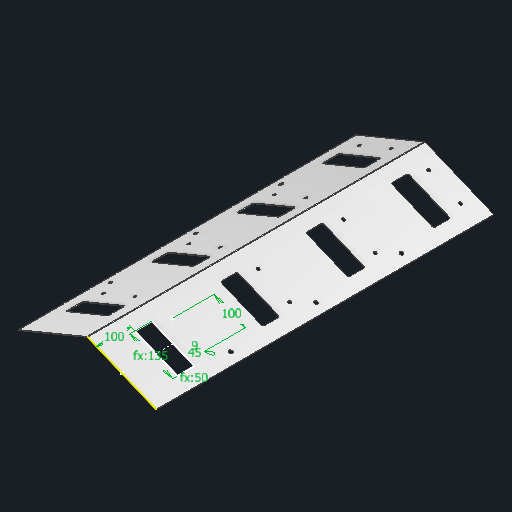
# Autodesk Inventor part: ASY DMF 010 cap №2 v2.1
Saved by Autodesk Inventor 2026.2 (Build 302298010, 298A)
## iProperties
Created: 2024-04-28
Part Number: ASY DMF 010 cap №2 v2.1
Material: Stainless Steel AISI 304
Document SubType Name: Sheet Metal
Designer: pokla
Stock Number: Барабан_Лист_Крышка
Density: 8 g/cm^3
Flat Pattern Width: 43.6215 cm
Flat Pattern Length: 98.85 cm
Flat Pattern Area: 4311.98 cm^2
Sheet Metal Rule: Default
Sheet Metal Width: 436,215 mm
Sheet Metal Length: 988,500 mm
Sheet Metal Area: 431198,146 mm^2
Appearance: Chrome - Satin
Author: pokla
Autodesk Inventor part; units mm, degrees
note: some values were not read from the file. Chosen so that the rebuilt part matches the saved one: flange form of "Plate4".
ref_plane "YZ Plane" through (0, 0, 0) normal (1, 0, 0) x (0, 1, 0)
ref_plane "XZ Plane" through (0, 0, 0) normal (0, 1, 0) x (-1, 0, 0)
ref_plane "XY Plane" through (0, 0, 0) normal (0, 0, 1) x (1, 0, 0)
sketch "Sketch1" plane through (0, 0, 0) normal (0, 0, 1) x (1, 0, 0)
  line L0 (-202.822219, 202.822219) -> (0, 286.833933) construction
  line L1 (0, 286.833933) -> (202.822219, 202.822219) construction
  line L2 (202.822219, 202.822219) -> (286.833933, 0) construction
  line L3 (286.833933, 0) -> (202.822219, -202.822219) construction
  line L4 (202.822219, -202.822219) -> (0, -286.833933) construction
  line L5 (0, -286.833933) -> (-202.822219, -202.822219) construction
  line L6 (-202.822219, -202.822219) -> (-286.833933, 0) construction
  line L7 (-286.833933, 0) -> (-202.822219, 202.822219) construction
  line L8 (1.530734, 286.199882) -> (201.990728, 203.166634)
  line L9 (-1.530734, 286.199882) -> (-201.990728, 203.166634)
  arc A0 (1.530734, 286.199882) -> (-1.530734, 286.199882) centre (0, 282.504364) ccw
  point P0 (0, 0)
  point P1 (0, 0)
  dimension "d46" = 530
  dimension "d47" = 0.9
  dimension "d48" = 4
  measures "d46" distance between parallel lines of L7 L3
  measures "d47" distance of L0.start L9.end
  measures "d48" radius of A0
contour flange "Contour Flange2" sketch "Sketch1" thickness 2 bend radius 2 width 988.5 along (0, 0, -1) mid plane no both sides no wall seen from (101.760731, 244.683258, 0) lies toward (-0.3826834, -0.9238795, 0) curves L8 A0 L9
bend "Bend4"
corner "Corner4"
sketch "Sketch14" plane through (1.530734, 286.199882, 0) normal (0.3826834, 0.9238795, 0) x (0.9238795, -0.3826834, 0)
  line L0 (175.988167, 150) -> (175.988167, 100)
  line L1 (175.988167, 100) -> (40.988167, 100)
  line L2 (40.988167, 100) -> (40.988167, 150)
  line L3 (40.988167, 150) -> (175.988167, 150)
  circle A0 centre (158.488167, 195) radius 4.5
  circle A1 centre (58.488167, 195) radius 4.5
  line L4 (108.488167, 100) -> (108.488167, 150) construction
  line L5 (216.976334, 0) -> (0, 0)
  point P0 (108.488167, 0)
  dimension "d163" = 9
  dimension "d164" = 135
  dimension "d165" = 50
  dimension "d166" = 45
  dimension "d167" = 100
  dimension "d171" = 100
  constraints: 10 end point, 3 midpoint, 2 centre point, 2 parallel, 1 perpendicular, 1 vertical alignment, 1 other
  measures "d163" diameter of A0
  measures "d164" distance of L2.end L0.start
  measures "d165" distance of L0.start L0.end
  measures "d166" distance from line of A0.centre L3
  measures "d167" distance of A1.centre A0.centre
  measures "d171" distance between parallel lines of L5 L1
extrude "Cut2" cut sketch "Sketch14" against normal through all
fillet "Fillet3" radius 5 4 edges at (39.0162, 269.5905, -150) (39.0162, 269.5905, -100) (163.7399, 217.9282, -100) (163.7399, 217.9282, -150)
pattern_linear "Rectangular Pattern7" count 4 spacing 250 along (0, 0, -1) of "Cut2", "Fillet3"
pattern_circular "Circular Pattern2" count 2 over 45 about axis through (0, 0, -10) along (0, 0, 1) of "Cut2", "Fillet3", "Rectangular Pattern7"
sketch "Sketch12" plane through (1.530734, 286.199882, 0) normal (0.3826834, 0.9238795, 0) x (0.9238795, -0.3826834, 0)
  circle A0 centre (189.129, 40.75) radius 5.5
  line L0 (0, 0) -> (0, 988.5)
  line L1 (216.976334, 0) -> (0, 0)
  line L2 (216.976334, 988.5) -> (0, 988.5)
  point P0 (108.10974, 0)
  dimension "d115" = 11
  dimension "d116" = 189.129
  dimension "d117" = 40.75
  constraints: 1 centre point
  measures "d115" diameter of A0
  measures "d116" distance from line of L0 A0.centre
  measures "d117" distance from line of L1 A0.centre
extrude "Extrusion5" [suppressed]
sketch "Sketch15" plane through (1.530734, 286.199882, 0) normal (0.3826834, 0.9238795, 0) x (0.9238795, -0.3826834, 0)
  circle A0 centre (189.129, 494.25) radius 5.5
  line L0 (0, 0) -> (0, 988.5) projected
  point P0 (108.10974, 0)
  point P1 (0, 494.25)
  dimension "d146" = 11
  dimension "d147" = 189.129
  constraints: 1 centre point, 1 horizontal alignment, 1 midpoint
  measures "d146" diameter of A0
  measures "d147" distance from line of L0 A0.centre
extrude "Extrusion8" cut sketch "Sketch15" against normal through all
pattern_linear "Rectangular Pattern6" count 3 spacing 250 along (0, 0, 1) of "Extrusion8" first direction both ways yes
mirror "Mirror5" about plane through (0, 0, 0) normal (1, 0, 0) of "Extrusion8", "Rectangular Pattern6"
equation "\"d46\" = Барабан_размер_по_плоскостям"
equation "\"d47\" = Барабан_отступ_развертки"
equation "\"d48\" = BendRadius + Thickness"
equation "\"d49\" = Thickness"
equation "\"d50\" = BendReliefWidth"
equation "\"d51\" = BendReliefDepth"
equation "\"d52\" = MinimumRemnant"
equation "\"d53\" = TransitionRadius"
equation "\"d55\" = BendRadius"
equation "\"d57\" = CornerReliefSize"
equation "\"d58\" = GapSize"
equation "\"d59\" = JacobiRadiusSize"
equation "\"BendRadius\" = Thickness"
equation "\"BendReliefWidth\" = Thickness"
equation "\"BendReliefDepth\" = 0.5 * Thickness"
equation "\"CornerReliefSize\" = 4 * Thickness"
equation "\"MinimumRemnant\" = 2 * Thickness"
equation "\"TransitionRadius\" = BendRadius"
equation "\"JacobiRadiusSize\" = BendRadius"
equation "\"GapSize\" = Thickness"
equation "\"Барабан_размер_по_плоскостям\" = 530"
equation "\"Барабан_отступ_развертки\" = 0.9"
equation "\"Thickness\" = 2"
body "Solid2"
